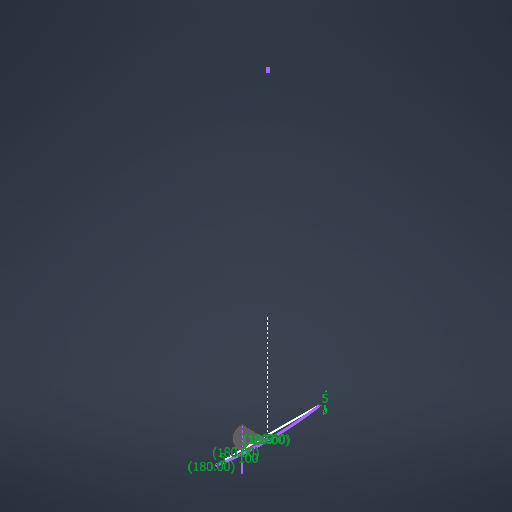
# Autodesk Inventor part: Pieza1
Saved by Autodesk Inventor 2026.1 (Build 301233020, 233B)
## iProperties
Created: 2026-05-16
Part Number: Pieza1
Material: Genérico
Document SubType Name: Modeling
Designer: USUARIO
Density: 1 g/cm^3
Appearance: Valor por defecto
Author: USUARIO
Autodesk Inventor part; units mm, degrees
ref_plane "YZ Plane" through (0, 0, 0) normal (1, 0, 0) x (0, 1, 0)
ref_plane "XZ Plane" through (0, 0, 0) normal (0, 1, 0) x (-1, 0, 0)
ref_plane "XY Plane" through (0, 0, 0) normal (0, 0, 1) x (1, 0, 0)
sketch "Boceto1" plane through (0, 0, 0) normal (1, 0, 0) x (0, 1, 0)
  line L0 (0, 0) -> (0, 125)
  line L1 (0, 0) -> (125, 0) construction
  line L2 (0, 0) -> (0, -125)
  line L3 (0, 0) -> (125, 0) construction
  line L4 (0, 0) -> (-20, 0)
  line L5 (0, 0) -> (20, 0) construction
  line L6 (0, 0) -> (500, 0) construction
  line L7 (0, 0) -> (-20, 0)
  line L8 (0, 0) -> (20, 0) construction
  line L9 (0, 0) -> (0, -246.4363)
  line L10 (0, 0) -> (246.4363, 0) construction
  line L11 (0, 0) -> (0, 250)
  line L12 (0, 0) -> (250, 0) construction
  arc A0 (0, 250) -> (0, -246.4363) centre (1530.2267, 1.7819) ccw
  line L13 (0, 125) -> (-100, 125)
  line L14 (0, 125) -> (100, 125) construction
  line L15 (0, 250) -> (-5, 250)
  line L16 (0, 250) -> (5, 250) construction
  line L17 (0, -246.4363) -> (-5, -246.4363)
  line L18 (-20, 0) -> (-23, 0)
  line L19 (-20, 0) -> (-17, 0) construction
  line L20 (-20, 0) -> (-25, 0)
  line L21 (-20, 0) -> (-15, 0) construction
  arc A1 (-5, 250) -> (-5, -246.4363) centre (1525.2267, 1.7819) ccw
  point P0 (-20.0963, 125)
  point P1 (-15.0963, 125)
  dimension "d14" = 100
  dimension "d15" = 180
  dimension "d16" = 5
  dimension "d17" = 180
  dimension "d18" = 5
  dimension "d19" = 3
  dimension "d20" = 180
  dimension "d21" = 5
  dimension "d22" = 180
  constraints: 44 end point, 17 horizontal, 10 equal length, 6 point on circle, 3 vertical, 2 centre point, 2 perpendicular
  measures "d14" distance of L0.end L13.end
  measures "d15" angle of L13 L14
  measures "d16" distance of L11.end L15.end
  measures "d17" angle of L15 L16
  measures "d18" distance of L9.end L17.end
  measures "d19" distance of L4.end L18.end
  measures "d20" angle of L18 L19
  measures "d21" distance of L4.end L20.end
  measures "d22" angle of L20 L21
revolve "Revolución1" add sketch "Boceto1" angle 90 about axis through (0, -20, 0) along (0, -1, 0) contours L18 L20 A1 L13 A0
fillet "Empalme1" radius 2 2 edges at (-88.3883, -15.0963, 88.3883) (-88.3883, -20.0963, 88.3883)
